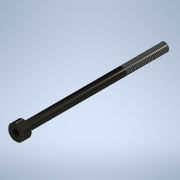
# Autodesk Inventor part: bolt_atas
Saved by Autodesk Inventor 2020 (Build 240168000, 168)
## iProperties
Created: 2020-02-02
Part Number: bolt_atas
Material: Generic
Document SubType Name: Modeling
Designer: Ferdi
Density: 1 g/cm^3
Appearance: Gunmetal
Author: Ferdi
Autodesk Inventor part; units mm, degrees
ref_plane "YZ Plane" through (0, 0, 0) normal (1, 0, 0) x (0, 1, 0)
ref_plane "XZ Plane" through (0, 0, 0) normal (0, 1, 0) x (-1, 0, 0)
ref_plane "XY Plane" through (0, 0, 0) normal (0, 0, 1) x (1, 0, 0)
sketch "Sketch1" plane through (0, 0, 0) normal (0, 0, 1) x (1, 0, 0)
  circle A0 centre (0, 0) radius 1.5
  circle A1 centre (0, 0) radius 2.75
  line L0 (1.4434, 0) -> (0.7217, -1.25)
  line L1 (0.7217, -1.25) -> (-0.7217, -1.25)
  line L2 (-0.7217, -1.25) -> (-1.4434, 0)
  line L3 (-1.4434, 0) -> (-0.7217, 1.25)
  line L4 (-0.7217, 1.25) -> (0.7217, 1.25)
  line L5 (0.7217, 1.25) -> (1.4434, 0)
  point P0 (1.4186, 0.4874)
  point P1 (1.4186, -0.4874)
  point P2 (1.1314, -0.9849)
  point P3 (0.2872, -1.4722)
  point P4 (-0.2872, -1.4722)
  point P5 (-1.1314, -0.9849)
  point P6 (-1.4186, -0.4874)
  point P7 (-1.4186, 0.4874)
  point P8 (-1.1314, 0.9849)
  point P9 (-0.2872, 1.4722)
  point P10 (0.2872, 1.4722)
  point P11 (1.1314, 0.9849)
  dimension "d2" = 3
  dimension "d3" = 5.5
  dimension "d15" = 2.5
  constraints: 12 end point, 2 centre point, 1 coincident, 13 other
  measures "d2" diameter of A0
  measures "d3" diameter of A1
  measures "d15" distance between parallel lines of L2 L5
extrude "Extrusion1" add sketch "Sketch1" against normal blind 50 contours A0 | L0 L1 L2 L3 L4 L5
extrude "Extrusion2" add sketch "Sketch1" along normal blind 3 contours A0 | A1
extrude "Extrusion3" add sketch "Sketch1" along normal blind 1 contours L0 L1 L2 L3 L4 L5
chamfer "Chamfer1" distance 0.3 angle 45 1 edges at (-2.75, 0, 3)
chamfer "Chamfer2" distance 0.2 angle 45 6 edges at (0, 1.25, 3) (-1.0825, 0.625, 3) (-1.0825, -0.625, 3) (0, -1.25, 3) (1.0825, -0.625, 3) (1.0825, 0.625, 3)
thread "Thread1" size "M3x0.5" class "6g" standard "ANSI Metric M Profile" length 15
body "Solid1"
